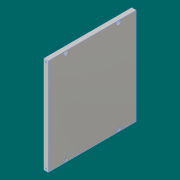
# Autodesk Inventor part: sides
Saved by Autodesk Inventor 2016 (Build 200138000, 138)
## iProperties
Created: 2015-10-13
Part Number: sides
Material: Aluminum 6061
Document SubType Name: Modeling
Designer: Sawaiz
Density: 2.7 g/cm^3
Appearance: Aluminum - Flat
Author: Sawaiz
Autodesk Inventor part; units mm, degrees
ref_plane "YZ Plane" through (0, 0, 0) normal (1, 0, 0) x (0, 1, 0)
ref_plane "XZ Plane" through (0, 0, 0) normal (0, 1, 0) x (-1, 0, 0)
ref_plane "XY Plane" through (0, 0, 0) normal (0, 0, 1) x (1, 0, 0)
sketch "Sketch1" plane through (0, 0, 0) normal (0, 1, 0) x (-1, 0, 0)
  line L0 (-60.071, 69.85) -> (60.071, 69.85)
  line L1 (60.071, 69.85) -> (60.071, -69.85)
  line L2 (60.071, -69.85) -> (-60.071, -69.85)
  line L3 (-60.071, -69.85) -> (-60.071, 69.85)
  line L4 (-60.071, 69.85) -> (60.071, -69.85) construction
  line L5 (60.071, 69.85) -> (-60.071, -69.85) construction
  point P0 (0, 0)
  dimension "d0" = 120.142
  dimension "d1" = 139.7
  constraints: 12 end point, 2 midpoint, 2 parallel, 1 horizontal, 1 perpendicular
  measures "d0" distance of L1.end L2.end
  measures "d1" distance of L0.end L1.end
extrude "Extrusion1" add sketch "Sketch1" along normal blind 6.35
sketch "Sketch9" plane through (60.071, 0, 69.85) normal (1, 0, 0) x (0, 0, -1)
  line L0 (139.7, 0) -> (0, 0) projected
  line L1 (139.7, 0) -> (139.7, 6.35) projected
  line L2 (0, 6.35) -> (139.7, 6.35) projected
  line L3 (0, 0) -> (0, 6.35) projected
  point P0 (69.85, 0)
  point P1 (3.175, 3.175)
  dimension "d45" = 3.175
  dimension "d46" = 3.175
  measures "d45" distance from line of L0 point (3.175, 3.175)
  measures "d46" distance from line of L3 point (3.175, 3.175)
hole "Hole3" at (60.071, 3.175, 66.675) direction (-1, 0, 0) diameter 2.156 depth 8.865 tip angle 118 thread size "4-40 UNC" class "2B" standard "ANSI Unified Screw Threads"
mirror "Mirror5" about plane through (0, 0, 0) normal (0, 0, 1) of "Hole3"
mirror "Mirror6" about plane through (0, 0, 0) normal (1, 0, 0) of "Hole3", "Mirror5"
sketch "Sketch10" plane through (0, 0, 0) normal (0, -1, 0) x (1, 0, 0)
  line L0 (60.071, 69.85) -> (-60.071, 69.85) projected
  line L1 (-60.071, 69.85) -> (-60.071, -69.85) projected
  line L2 (-60.071, -69.85) -> (60.071, -69.85) projected
  line L3 (60.071, -69.85) -> (60.071, 69.85) projected
  line L4 (21.1773, -65.0875) -> (22.7648, -65.0875)
  line L5 (22.7648, -65.0875) -> (22.7648, 65.0875)
  line L6 (22.7648, 65.0875) -> (21.1773, 65.0875)
  line L7 (21.1773, 65.0875) -> (21.1773, -65.0875)
  point P0 (0, 0)
  dimension "d54" = 1.5875
  dimension "d55" = 37.3062
  dimension "d56" = 4.7625
  dimension "d57" = 4.7625
  constraints: 8 end point, 2 parallel, 1 horizontal, 1 perpendicular
  measures "d54" distance between parallel lines of L5 L7
  measures "d55" distance between parallel lines of L3 L5
  measures "d56" distance between parallel lines of L0 L6
  measures "d57" distance between parallel lines of L2 L4
extrude "Extrusion6" cut sketch "Sketch10" against normal blind 1.5875 contours L7 L6 L5 L4
fillet "Fillet2" radius 0.7937 4 edges at (22.7648, 0.7937, 65.0875) (21.1773, 0.7937, 65.0875) (22.7648, 0.7937, -65.0875) (21.1773, 0.7937, -65.0875)
sketch "Sketch11" plane through (0, 6.35, 0) normal (0, 1, 0) x (1, 0, 0)
  line L0 (-60.071, -69.85) -> (60.071, -69.85) projected
  line L1 (60.071, -69.85) -> (60.071, 69.85) projected
  line L2 (60.071, 69.85) -> (-60.071, 69.85) projected
  line L3 (-60.071, 69.85) -> (-60.071, -69.85) projected
  point P0 (0, 0)
  point P1 (34.671, -66.675)
  dimension "d61" = 25.4
  dimension "d62" = 3.175
  measures "d61" distance from line of L1 point (34.671, -66.675)
  measures "d62" distance from line of L0 point (34.671, -66.675)
hole "Hole4" at (34.671, 6.35, 66.675) direction (0, -1, 0) diameter 3.264 end through all countersink diameter 5.715 countersink angle 82 clearance for "Flat Head Machine Screw (82)" size "#4" standard "Ansi Unified Screw Threads"
mirror "Mirror7" about plane through (0, 0, 0) normal (1, 0, 0) of "Hole4"
mirror "Mirror8" about plane through (0, 0, 0) normal (0, 0, 1) of "Hole4", "Mirror7"
equation "\"d0\" = depth"
equation "\"d1\" = height + 2 * plasticThickness"
equation "\"d2\" = caseThickness"
equation "\"d45\" = 0.5 * caseThickness"
equation "\"d46\" = 0.5 * caseThickness"
equation "\"d55\" = aerogelHolderDepth"
equation "\"d58\" = 0.25 * caseThickness"
equation "\"d61\" = 4 * caseThickness"
equation "\"d62\" = 0.5 * caseThickness"
equation "\"acrylicThickness\" = 9.525"
equation "\"depth\" = 120.142"
equation "\"height\" = 127"
equation "\"fresnelThickness\" = 0.1"
equation "\"focalLength\" = 76.2"
equation "\"centerThickness\" = 1.524"
equation "\"sensorHolderDepth\" = 19.05"
equation "\"internalAcrylicThickness\" = 6.35"
equation "\"frameAcrylicThickness\" = 9.525"
equation "\"width\" = 127"
equation "\"mirrorAngle\" = 5deg"
equation "\"detectorWidth\" = 52"
equation "\"detectorHeight\" = 52"
equation "\"mirrorThickness\" = 3.175"
equation "\"ior\" = 1.49"
equation "\"fresnelAngle\" = 90deg"
equation "\"fresnelEffectiveDiameter\" = 152.4"
equation "\"oRingWidth\" = 1.5875"
equation "\"aerogelClearence\" = 3.175"
equation "\"backplanePCBHeight\" = 76.2"
equation "\"backplaneHoleOffsett\" = 6.35"
equation "\"backplanePCBWidth\" = 76.2"
equation "\"backplanePostionOffsett\" = 12.7"
equation "\"moduleSlotClearence\" = 0.79375"
equation "\"plasticThickness\" = 6.35"
equation "\"aerogelHolderDepth\" = 37.30625"
equation "\"caseThickness\" = 6.35"
body "Solid1"
